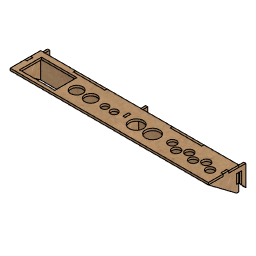
Prateleira para Bancada de Eletrônica (Autodesk Fusion 360 archive; units mm, degrees)
design "Suporte de Ferramentas"
Autodesk Fusion 360 part; units mm, degrees
note: some values were not read from the file. Set by a fixed rule: which face or edge a step refers to.
sketch "Sketch1" plane through (0, 0, 0) normal (0, 1, 0) x (1, 0, 0)
  line L0 (-140, -30) -> (140, -30)
  line L1 (140, -30) -> (140, 0)
  line L2 (140, 0) -> (-140, 0)
  line L3 (-140, 0) -> (-140, -30)
  dimension "d1" = 280
  dimension "d5" = 30
  constraint horizontal L0
  constraint vertical L1
  constraint horizontal L2
  constraint vertical L3
  constraint midpoint origin L2
  measures "d1" distance of L0.start L0.end
  measures "d5" distance of L0.start L2.end
extrude "Extrude1" add sketch "Sketch1" along normal blind 3 makes body 1
sketch "Sketch2" plane through (140, 0, 0) normal (1, 0, 0) x (0, 1, 0)
  line L0 (0, 30) -> (0, 0)
  line L1 (0, 0) -> (3, 0)
  line L2 (3, 0) -> (3, 30)
  line L3 (3, 30) -> (0, 30)
  line L4 (0, 30) -> (-40, 30)
  line L5 (0, 23.7831) -> (3, 23.7831)
  line L6 (3, 23.7831) -> (3, 10.8609)
  line L7 (3, 10.8609) -> (0, 10.8609)
  line L8 (0, 10.8609) -> (0, 23.7831)
  line L9 (3, 30) -> (7, 30)
  line L10 (7, 30) -> (7, 23.7831)
  line L11 (7, 23.7831) -> (3, 23.7831)
  line L12 (3, 23.7831) -> (3, 30)
  line L13 (7, 30) -> (13, 30)
  line L14 (13, 30) -> (13, 0)
  line L15 (7, 6.72) -> (7, 30)
  line L16 (-19.0587, 30) -> (-11.052, 30)
  line L17 (-11.052, 30) -> (-11.052, 33)
  line L18 (-11.052, 33) -> (-19.0587, 33)
  line L19 (-19.0587, 33) -> (-19.0587, 30)
  line L20 (13, 0) -> (7, 6.72)
  line L21 (0, 0) -> (13, 0) construction
  line L22 (-40, 30) -> (0, 0)
  dimension "d10" = 40
  dimension "d11" = 4
  dimension "d48" = 3
  dimension "d69" = 6
  constraint coincident L0.start L3.end
  constraint perpendicular L0 L4
  constraint horizontal L5
  constraint vertical L6
  constraint horizontal L7
  constraint vertical L8
  constraint coincident L2 L6.end
  constraint coincident L0 L5.start
  constraint horizontal L9
  constraint vertical L10
  constraint horizontal L11
  constraint vertical L12
  constraint coincident L2.end L3.start
  constraint horizontal L13
  constraint vertical L14
  constraint vertical L15
  constraint horizontal L16
  constraint vertical L17
  constraint horizontal L18
  constraint vertical L19
  constraint coincident L4 L16.start
  constraint coincident L0.end L1.start
  constraint perpendicular L0 L21
  measures "d10" distance of L0.start L4.end
  measures "d11" distance of L2.end L9.end
  measures "d48" distance of L16.start L18.end
  measures "d69" distance of L9.end L13.end
extrude "Extrude2" add sketch "Sketch2" against normal blind 3 separate body contours L0 L2 L3 L5 L12 | L0 L4 L8 L16 L22 | L2 L9 L10 L11 L12 L15 | L4 L16 L17 L18 L19 | L0 L1 L2 L7 | L10 L13 L14 L15 L20 makes body 2
pattern_linear "R-Pattern1" count 3 spacing 138.5 along (-1, 0, 0) of bodies 2 makes body 3 at (1.5, -19.6862, 20) makes body 4 at (-137, -19.6862, 20)
combine "Combine1" operation cut target body 1 tool bodies 3 2 4 keep tools
sketch "Suporte" plane through (137, 0, 0) normal (-1, 0, 0) x (0, -1, 0)
  line L0 (40, 30) -> (19.0587, 30)
  line L1 (-13, 30) -> (-13, 0)
  line L2 (-7, 6.72) -> (-7, 23.7831)
  line L3 (-7, 23.7831) -> (0, 23.7831)
  line L4 (0, 23.7831) -> (0, 10.8609)
  line L5 (0, 10.8609) -> (-3, 10.8609)
  line L6 (-3, 10.8609) -> (-3, 0)
  line L7 (-3, 0) -> (0, 0)
  line L8 (19.0587, 30) -> (19.0587, 33)
  line L9 (19.0587, 33) -> (11.052, 33)
  line L10 (11.052, 33) -> (11.052, 30)
  line L11 (0, 0) -> (40, 30)
  line L12 (11.052, 30) -> (-13, 30)
  line L13 (-13, 0) -> (-7, 6.72)
sketch "Sketch4" plane through (0, 0, 30) normal (0, 0, 1) x (-1, 0, 0)
  line L0 (-140, -13) -> (-137, -13)
  line L1 (-1.5, -13) -> (1.5, -13)
  line L2 (140, -3) -> (-139.9985, -3)
  line L3 (-139.9985, -3) -> (-139.9985, 40)
  line L4 (-139.9985, 40) -> (140, 40)
  line L5 (140, 40) -> (140, -3)
  line L6 (140, 20) -> (-140, 20) construction
  circle A0 centre (-125.871, 23.3241) radius 5.75
  circle A1 centre (-41.1601, 20) radius 10
  circle A2 centre (-18.1601, 20) radius 10
  circle A3 centre (13.0751, 20) radius 5
  circle A4 centre (26.0751, 20) radius 5
  line L7 (81.3069, 35.5) -> (131.3069, 35.5)
  line L8 (131.3069, 35.5) -> (131.3069, 4.5)
  line L9 (131.3069, 4.5) -> (81.3069, 4.5)
  line L10 (81.3069, 4.5) -> (81.3069, 35.5)
  line L11 (81.3069, 35.5) -> (131.3069, 4.5) construction
  line L12 (131.3069, 35.5) -> (81.3069, 4.5) construction
  line L13 (140, 0) -> (140, 40)
  line L14 (137, 0) -> (140, 0) construction
  line L15 (-1.5, -3) -> (-137, -3)
  line L16 (-1.5, 0) -> (-137, 0)
  line L17 (137, -3) -> (1.5, -3)
  line L18 (137, 0) -> (1.5, 0)
  line L19 (137, -13) -> (140, -13)
  line L20 (90.7932, -3) -> (46.2097, -3)
  line L21 (46.2097, -3) -> (46.2097, 0)
  line L22 (46.2097, 0) -> (90.7932, 0)
  line L23 (90.7932, 0) -> (90.7932, -3)
  line L24 (0.0007, -3) -> (0.0007, 40) construction
  line L25 (-90.7917, -0.0001) -> (-90.7917, -3.0001)
  line L26 (-90.7917, -3.0001) -> (-46.2082, -3.0001)
  line L27 (-46.2082, -3.0001) -> (-46.2082, -0.0001)
  line L28 (-46.2082, -0.0001) -> (-90.7917, -0.0001)
  line L29 (90.7932, -1.5) -> (137.0021, -1.5) construction
  line L30 (46.2097, -1.5) -> (0.0007, -1.5) construction
  circle A5 centre (46.0653, 20) radius 8.5
  circle A6 centre (66.0653, 20) radius 8.5
  line L31 (-140, 11.052) -> (-140, -13)
  line L32 (-137, -13) -> (-137, 11.052)
  line L33 (-137, 11.052) -> (-140, 11.052)
  line L34 (-1.5, 11.052) -> (-1.5, -13)
  line L35 (1.5, -13) -> (1.5, 11.052)
  line L36 (1.5, 11.052) -> (-1.5, 11.052)
  line L37 (137, 11.052) -> (137, -13)
  line L38 (140, -13) -> (140, 11.052)
  line L39 (140, 11.052) -> (137, 11.052)
  line L40 (-125.871, 23.3241) -> (-125.871, 20) construction
  circle A7 centre (-113.871, 16.6759) radius 5.75
  line L41 (-113.871, 16.6759) -> (-125.871, 23.3241) construction
  line L42 (-113.871, 16.6759) -> (-125.871, 16.6759) construction
  circle A8 centre (-89.871, 16.6759) radius 5.75
  circle A9 centre (-101.871, 23.3241) radius 5.75
  circle A10 centre (-65.871, 16.6759) radius 5.75
  circle A11 centre (-77.871, 23.3241) radius 5.75
  line L43 (-125.871, 20) -> (-125.871, 16.6759) construction
  line L44 (0, 0) -> (0, 0)
  point P0 (106.3069, 20)
  point P1 (140, 40)
  dimension "d22" = 11.5
  dimension "d27" = 20
  dimension "d30" = 23
  dimension "d31" = 0
  dimension "d32" = 10
  dimension "d35" = 13
  dimension "d36" = 0
  dimension "d37" = 50
  dimension "d38" = 31
  dimension "d43" = 17
  dimension "d46" = 20
  dimension "d47" = 0
  dimension "d63" = 11.5
  dimension "d72" = 24
  dimension "d73" = 0
  dimension "d76" = 12
  constraint horizontal L2
  constraint vertical L3
  constraint horizontal L4
  constraint vertical L5
  constraint coincident L6 A1.centre
  constraint coincident L6 A3.centre
  constraint horizontal L7
  constraint perpendicular L7 L8
  constraint parallel L7 L9
  constraint parallel L8 L10
  constraint coincident L11 P0
  constraint coincident L12 P0
  constraint coincident L6 P0
  constraint midpoint L6.start L13
  constraint horizontal L6
  constraint coincident L5 L13.start
  constraint horizontal L14
  constraint collinear L2 L17
  constraint coincident L14.start L18.start
  constraint horizontal L20
  constraint vertical L21
  constraint horizontal L22
  constraint vertical L23
  constraint coincident L18 L21.end
  constraint coincident L2 L20.start
  constraint coincident L17 L20.start
  constraint midpoint L2 L24.start
  constraint symmetric L20.start L24 L25.end
  constraint symmetric L20.end L24 L26.end
  constraint symmetric L21.end L24 L27.end
  constraint symmetric L22.end L24 L25.start
  constraint midpoint L23 L29.start
  constraint midpoint L21 L30.start
  constraint coincident L24 L30.end
  constraint perpendicular L24 L30
  constraint equal L29 L30
  constraint coincident L6 A5.centre
  constraint coincident A0.centre L40.start
  constraint coincident L6 L40.end
  constraint perpendicular L6 L40
  constraint coincident A7.centre L41.start
  constraint perpendicular L40 L42
  constraint perpendicular L42 L43
  constraint equal L40 L43
  constraint coincident P1 L4.end
  measures "d22" diameter of A0
  measures "d27" diameter of A1
  measures "d32" diameter of A3
  measures "d37" distance of L8.end L9.end
  measures "d38" distance of L7.end L8.end
  measures "d43" diameter of A5
  measures "d63" diameter of A7
  measures "d76" distance of A7.centre L42.end
extrude "Extrude7" add 2 faces at (46.6667, 1, 30) (-91.8333, 2, 30) along direction (0, 0, 1) blind 3 on bodies 1 bodies 1
extrude "Extrude4" add sketch "Sketch4" along normal blind 3 separate body contours L2 L3 L31 L32 L33 | L2 L15 L16 L25 L32 | L3 L4 L5 L13 L16 L18 L22 L28 L32 L33 L34 L35 L36 L37 L39 | L2 L15 L16 L27 L34 | L2 L34 L35 L36 | L2 L5 L13 L37 L38 L39 | L2 L17 L18 L21 L35 | L2 L17 L18 L23 L37 makes body 5
sketch "Sketch5" plane through (0, 0, 33) normal (0, 0, 1) x (-1, 0, 0)
  circle A0 centre (-41.1601, 20) radius 10
  circle A1 centre (13.0751, 20) radius 5
  circle A2 centre (26.0751, 20) radius 5
  circle A3 centre (-125.871, 23.3241) radius 5.75
  line L0 (131.3069, 4.5) -> (81.3069, 4.5)
  line L1 (81.3069, 4.5) -> (81.3069, 35.5)
  line L2 (81.3069, 35.5) -> (131.3069, 35.5)
  line L3 (131.3069, 35.5) -> (131.3069, 4.5)
  circle A4 centre (-18.1601, 20) radius 10
  line L4 (46.2097, -3) -> (46.2097, 0)
  line L5 (46.2097, 0) -> (90.7932, 0)
  line L6 (90.7932, 0) -> (90.7932, -3)
  line L7 (90.7932, -3) -> (140, -3)
  line L8 (140, -3) -> (140, 40)
  line L9 (140, 40) -> (-139.9985, 40)
  line L10 (-139.9985, 40) -> (-139.9985, -3)
  line L11 (-139.9985, -3) -> (-90.7917, -3)
  line L12 (-90.7917, -3) -> (-90.7917, -0.0001)
  line L13 (-90.7917, -0.0001) -> (-46.2082, -0.0001)
  line L14 (-46.2082, -0.0001) -> (-46.2082, -3)
  line L15 (-46.2082, -3) -> (46.2097, -3)
  circle A5 centre (46.0653, 20) radius 8.5
  circle A6 centre (66.0653, 20) radius 8.5
  circle A7 centre (-113.871, 16.6759) radius 5.75
  circle A8 centre (-101.871, 23.3241) radius 5.75
  circle A9 centre (-89.871, 16.6759) radius 5.75
  circle A10 centre (-65.871, 16.6759) radius 5.75
  circle A11 centre (-77.871, 23.3241) radius 5.75
combine "Combine2" operation cut target body 5 tool bodies 3 4 2 keep tools
combine "Combine4" operation cut target body 1 tool bodies 5 keep tools
sketch "Gancho" plane through (-140, 0, 0) normal (-1, 0, 0) x (0, -1, 0)
  line L0 (0, 23.7831) -> (0, 10.8609)
  line L1 (0, 10.8609) -> (-3, 10.8609)
  line L2 (-3, 10.8609) -> (-3, 0)
  line L3 (-3, 0) -> (0, 0)
  line L4 (0, 0) -> (40, 30)
  line L5 (40, 30) -> (19.0587, 30)
  line L6 (19.0587, 30) -> (19.0587, 33)
  line L7 (19.0587, 33) -> (11.052, 33)
  line L8 (11.052, 33) -> (11.052, 30)
  line L9 (11.052, 30) -> (-13, 30)
  line L10 (-13, 30) -> (-13, 0)
  line L11 (-13, 0) -> (-7, 6.72)
  line L12 (-7, 6.72) -> (-7, 23.7831)
  line L13 (-7, 23.7831) -> (0, 23.7831)
sketch "Traseira" plane through (0, 3, 0) normal (0, 1, 0) x (-1, 0, 0)
  line L0 (-90.7917, 30) -> (-137, 30)
  line L1 (-137, 30) -> (-137, 23.7831)
  line L2 (-137, 23.7831) -> (-140, 23.7831)
  line L3 (-140, 23.7831) -> (-140, 10.8609)
  line L4 (-140, 10.8609) -> (-137, 10.8609)
  line L5 (-137, 10.8609) -> (-137, 0)
  line L6 (-137, 0) -> (-1.5, 0)
  line L7 (-1.5, 0) -> (-1.5, 10.8609)
  line L8 (-1.5, 10.8609) -> (1.5, 10.8609)
  line L9 (1.5, 10.8609) -> (1.5, 0)
  line L10 (1.5, 0) -> (137, 0)
  line L11 (137, 0) -> (137, 10.8609)
  line L12 (137, 10.8609) -> (140, 10.8609)
  line L13 (140, 10.8609) -> (140, 23.7831)
  line L14 (140, 23.7831) -> (137, 23.7831)
  line L15 (137, 23.7831) -> (137, 30)
  line L16 (137, 30) -> (90.7932, 30)
  line L17 (90.7932, 30) -> (90.7932, 33)
  line L18 (90.7932, 33) -> (46.2097, 33)
  line L19 (46.2097, 33) -> (46.2097, 30)
  line L20 (46.2097, 30) -> (1.5, 30)
  line L21 (1.5, 30) -> (1.5, 23.7831)
  line L22 (1.5, 23.7831) -> (-1.5, 23.7831)
  line L23 (-1.5, 23.7831) -> (-1.5, 30)
  line L24 (-1.5, 30) -> (-46.2082, 30)
  line L25 (-46.2082, 30) -> (-46.2082, 33)
  line L26 (-46.2082, 33) -> (-90.7917, 33)
  line L27 (-90.7917, 33) -> (-90.7917, 30)
sketch "Topo" plane through (0, 0, 33) normal (0, 0, 1) x (-1, 0, 0)
  line L0 (-137, 11.052) -> (-139.9985, 11.052)
  line L1 (-139.9985, 11.052) -> (-139.9985, -3)
  line L2 (-139.9985, -3) -> (-90.7917, -3)
  line L3 (-90.7917, -3) -> (-90.7917, -0.0001)
  line L4 (-90.7917, -0.0001) -> (-46.2082, -0.0001)
  line L5 (-46.2082, -0.0001) -> (-46.2082, -3)
  line L6 (-46.2082, -3) -> (46.2097, -3)
  line L7 (46.2097, -3) -> (46.2097, 0)
  line L8 (46.2097, 0) -> (90.7932, 0)
  line L9 (90.7932, 0) -> (90.7932, -3)
  line L10 (90.7932, -3) -> (140, -3)
  line L11 (140, -3) -> (140, 11.052)
  line L12 (140, 11.052) -> (137, 11.052)
  line L13 (137, 11.052) -> (137, 19.0587)
  line L14 (137, 19.0587) -> (140, 19.0587)
  line L15 (140, 19.0587) -> (140, 40)
  line L16 (140, 40) -> (-139.9985, 40)
  line L17 (-139.9985, 40) -> (-139.9985, 19.0587)
  line L18 (-139.9985, 19.0587) -> (-137, 19.0587)
  line L19 (-137, 19.0587) -> (-137, 11.052)
  circle A0 centre (-125.871, 23.3241) radius 5.75
  circle A1 centre (-101.871, 23.3241) radius 5.75
  circle A2 centre (-89.871, 16.6759) radius 5.75
  circle A3 centre (46.0653, 20) radius 8.5
  circle A4 centre (66.0653, 20) radius 8.5
  circle A5 centre (-113.871, 16.6759) radius 5.75
  line L20 (131.3069, 4.5) -> (81.3069, 4.5)
  line L21 (81.3069, 4.5) -> (81.3069, 35.5)
  line L22 (81.3069, 35.5) -> (131.3069, 35.5)
  line L23 (131.3069, 35.5) -> (131.3069, 4.5)
  circle A6 centre (26.0751, 20) radius 5
  circle A7 centre (13.0751, 20) radius 5
  circle A8 centre (-18.1601, 20) radius 10
  circle A9 centre (-41.1601, 20) radius 10
  circle A10 centre (-77.871, 23.3241) radius 5.75
  circle A11 centre (-65.871, 16.6759) radius 5.75
  line L24 (-1.5, 19.0587) -> (1.5, 19.0587)
  line L25 (1.5, 19.0587) -> (1.5, 11.052)
  line L26 (1.5, 11.052) -> (-1.5, 11.052)
  line L27 (0, 0) -> (0, 0)
equation "d1 = comprimentoSuporte"
equation "comprimentoSuporte = 280 mm"
equation "alturaSuporte = 30 mm"
equation "espessuraMaterial = 3 mm"
equation "d5 = alturaSuporte"
equation "d6 = espessuraMaterial"
equation "larguraSuporte = 40 mm"
equation "d10 = larguraSuporte"
equation "d11 = espessuraGradeado"
equation "d13 = -espessuraMaterial"
equation "d19 = comprimentoSuporte - espessuraMaterial"
equation "espessuraGradeado = 4 mm"
equation "d39 = espessuraMaterial"
equation "d48 = espessuraMaterial"
equation "d63 = d22"
equation "d72 = d76 * 2"
equation "d77 = espessuraMaterial"
